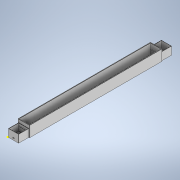
# Autodesk Inventor part: DRAINAGE
Saved by Autodesk Inventor 2022 (Build 260153000, 153)
## iProperties
Created: 2022-03-28
Part Number: DRAINAGE
Material: Generic
Document SubType Name: Modeling
Designer: minali
Density: 1 g/cm^3
Appearance: Default
Author: minali
Autodesk Inventor part; units mm, degrees
ref_plane "YZ Plane" through (0, 0, 0) normal (1, 0, 0) x (0, 1, 0)
ref_plane "XZ Plane" through (0, 0, 0) normal (0, 1, 0) x (-1, 0, 0)
sketch "Sketch1" plane through (0, 0, 0) normal (0, 0, 1) x (1, 0, 0)
  line L0 (0, 150) -> (0, 0)
  line L1 (0, 150) -> (10, 150)
  line L2 (10, 150) -> (10, 10)
  line L3 (10, 10) -> (150, 10)
  line L4 (150, 10) -> (150, 150)
  line L5 (150, 150) -> (160, 150)
  line L6 (160, 150) -> (160, 0)
  line L7 (160, 0) -> (0, 0)
  dimension "d0" = 10
  dimension "d1" = 10
  dimension "d2" = 150
  dimension "d3" = 160
  dimension "d4" = 10
  constraints: 16 end point, 5 perpendicular, 2 vertical, 1 horizontal
  measures "d0" distance of L0.start L1.end
  measures "d1" distance of L4.end L5.end
  measures "d2" distance of L0.start L0.end
  measures "d3" distance of L6.end L0.end
  measures "d4" distance between parallel lines of L7 L3
extrude "Extrusion1" add sketch "Sketch1" along normal blind 1800
sketch "Sketch2" plane through (0, 0, 1800) normal (0, 0, 1) x (1, 0, 0)
  line L0 (0, 0) -> (160, 0) projected
  line L1 (160, 0) -> (160, 150) projected
  line L2 (0, 0) -> (160, 0)
  line L3 (160, 0) -> (160, 150)
  line L4 (160, 150) -> (0, 150)
  line L5 (0, 150) -> (0, 0)
  constraints: 8 end point, 2 parallel, 1 horizontal, 1 perpendicular
extrude "Extrusion2" add sketch "Sketch2" along normal blind 10
sketch "Sketch3" plane through (0, 0, 1810) normal (0, 0, 1) x (1, 0, 0)
  line L0 (0, 0) -> (160, 0) projected
  line L1 (80, 0) -> (80, 70)
  line L2 (10, 10) -> (10, 150) projected
  line L3 (150, 150) -> (150, 10) projected
  line L4 (10, 70) -> (150, 70)
  line L5 (150, 70) -> (150, 80)
  line L6 (150, 80) -> (10, 80)
  line L7 (10, 80) -> (10, 70)
  point P0 (10, 80)
  dimension "d9" = 70
  dimension "d10" = 10
  constraints: 10 end point, 2 midpoint, 2 parallel, 1 horizontal, 1 perpendicular, 1 point on line, 1 vertical
  measures "d9" distance of L1.start L1.end
  measures "d10" distance between parallel lines of L4 L6
extrude "Extrusion3" cut sketch "Sketch3" against normal blind 10
sketch "Sketch4" plane through (0, 0, 1810) normal (0, 0, 1) x (1, 0, 0)
  line L0 (150, 150) -> (150, 80) projected
  line L1 (10, 0) -> (150, 0)
  line L2 (150, 0) -> (150, 108.9541)
  line L3 (150, 108.9541) -> (10, 108.9541)
  line L4 (10, 108.9541) -> (10, 0)
  point P0 (0, 0)
  constraints: 8 end point, 2 parallel, 1 horizontal, 1 perpendicular, 1 point on line
extrude "Extrusion4" add sketch "Sketch4" along normal blind 140
sketch "Sketch5" plane through (10, 108.9541, 1810) normal (0, 1, 0) x (1, 0, 0)
  point P0 (-10, 1810)
sketch "Sketch6" plane through (0, 0, 1950) normal (0, 0, 1) x (1, 0, 0)
  point P0 (0, 0)
sketch "Sketch7" plane through (10, 108.9541, 1810) normal (0, 1, 0) x (1, 0, 0)
  line L0 (5, -5) -> (135, -5)
  line L1 (135, -5) -> (135, -135)
  line L2 (135, -135) -> (5, -135)
  line L3 (5, -135) -> (5, -5)
  line L4 (0, 0) -> (140, 0) projected
  line L5 (140, 0) -> (140, -140) projected
  line L6 (140, -140) -> (0, -140) projected
  line L7 (0, 0) -> (0, -140) projected
  point P0 (-10, 1810)
  dimension "d15" = 5
  dimension "d16" = 5
  dimension "d17" = 5
  dimension "d18" = 5
  constraints: 8 end point, 2 parallel, 1 horizontal, 1 perpendicular
  measures "d15" distance between parallel lines of L4 L0
  measures "d16" distance between parallel lines of L5 L1
  measures "d17" distance between parallel lines of L6 L2
  measures "d18" distance between parallel lines of L7 L3
extrude "Extrusion5" cut sketch "Sketch7" against normal blind 98.954 contours L0 L1 L2 L3
sketch "Sketch8" plane through (0, 0, 1950) normal (0, 0, 1) x (1, 0, 0)
  circle A0 centre (80, 29.8763) radius 10
  point P0 (0, 0)
  dimension "d21" = 20
  constraints: 1 centre point
  measures "d21" diameter of A0
extrude "Extrusion6" cut sketch "Sketch8" against normal blind 5
sketch "Sketch9" plane through (15, 108.9541, 1815) normal (0, 0, 1) x (1, 0, 0)
  line L0 (-5, -38.9541) -> (135, -38.9541) projected
  line L1 (135, -28.9541) -> (-5, -28.9541) projected
  line L2 (135, -38.9541) -> (-5, -38.9541)
  line L3 (-5, -38.9541) -> (-5, -28.9541)
  line L4 (-5, -28.9541) -> (135, -28.9541)
  line L5 (135, -28.9541) -> (135, -38.9541)
  point P0 (-15, -108.9541)
  constraints: 8 end point, 2 parallel, 1 horizontal, 1 perpendicular
extrude "Extrusion7" cut sketch "Sketch9" against normal blind 5
ref_plane "Work Plane1" through (0, 0, 900) normal (0, 0, -1) x (-1, 0, 0)
mirror "Mirror1" about plane through (0, 0, 900) normal (0, 0, -1)
mirror "Mirror2" about plane through (0, 0, 900) normal (0, 0, -1) of "Extrusion4", "Extrusion3", "Extrusion1", "Extrusion6", "Extrusion5", "Extrusion2"
sketch "Sketch10" plane through (10, 0, 1810) normal (-1, 0, 0) x (0, 0, 1)
  line L0 (5, 80) -> (5, 70) projected
  line L1 (5, 70) -> (0, 70) projected
  line L2 (5, 80) -> (0, 80)
  line L3 (0, 80) -> (0, 70)
  line L4 (0, 70) -> (5, 70)
  line L5 (5, 70) -> (5, 80)
  point P0 (-1810, 0)
  constraints: 8 end point, 2 parallel, 1 horizontal, 1 perpendicular
extrude "Extrusion8" add sketch "Sketch10" against normal blind 5
sketch "Sketch11" plane through (150, 0, 1810) normal (1, 0, 0) x (0, 0, -1)
  line L0 (-5, 108.9541) -> (-5, 80) projected
  line L1 (0, 70) -> (0, 80) projected
  line L2 (-5, 80) -> (0, 80)
  line L3 (0, 80) -> (0, 70)
  line L4 (0, 70) -> (-5, 70)
  line L5 (-5, 70) -> (-5, 80)
  point P0 (1810, 0)
  constraints: 8 end point, 2 parallel, 1 horizontal, 1 perpendicular
extrude "Extrusion9" add sketch "Sketch11" against normal blind 5
sketch "Sketch12" plane through (145, 108.9541, -15) normal (0, 0, -1) x (-1, 0, 0)
  line L0 (135, -38.9541) -> (-5, -38.9541) projected
  line L1 (130, -29.6689) -> (0, -29.6689)
  line L2 (0, -29.6689) -> (0, -38.9541)
  line L3 (0, -38.9541) -> (130, -38.9541)
  line L4 (130, -38.9541) -> (130, -29.6689)
  point P0 (145, -108.9541)
  point P1 (130, 0)
  point P2 (0, 0)
  dimension "d31" = 0
  dimension "d32" = 0
  constraints: 8 end point, 2 parallel, 1 horizontal, 1 perpendicular, 1 point on line
  measures "d31" distance from line of point (130, 0) L4
  measures "d32" distance from line of point (0, 0) L2
extrude "Extrusion10" cut sketch "Sketch12" against normal blind 5
fillet "Fillet1" radius 2 20 edges at (160, 150, 900) (150, 150, 900) (10, 150, 900) (0, 150, 900) (0, 0, 900) (0, 75, -10) (160, 75, -10) (160, 0, 900) (155, 0, -10) (5, 0, -10) (10, 54.4771, -150) (150, 54.4771, -150) (80, 0, -150) (80, 108.9541, -150) (10, 108.9541, -80) (15, 108.9541, -80) (145, 108.9541, -80) (150, 108.9541, -80) (80, 150, -10) (80, 150, 0)
fillet "Fillet2" radius 2 25 edges at (0.5858, 149.4142, 1810) (0, 75, 1810) (0.5858, 0.5858, 1810) (6, 0, 1810) (159.4142, 149.4142, 1810) (160, 75, 1810) (159.4142, 0.5858, 1810) (154, 0, 1810) (80, 150, 1810) (9, 150, 1800) (80, 108.9541, 1815) (15, 108.9541, 1880) (10, 108.9541, 1880) (80, 108.9541, 1950) (80, 108.9541, 1945) (150, 108.9541, 1880) (145, 108.9541, 1880) (80, 0, 1950) (150, 54.4771, 1950) (150, 0, 1880) (10, 54.4771, 1950) (10, 0, 1880) (80, 10.0001, 1815) (80, 70, 1815) (80, 80, 1815)
ref_plane "Work Plane2" through (0, 0, 900) normal (0, 0, -1) x (-1, 0, 0)
body "Solid1"
